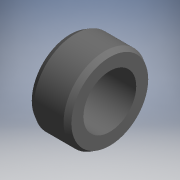
# Autodesk Inventor part: 189652 ZBH-5
Saved by Autodesk Inventor 2017.3 (Build 213256000, 256)
## iProperties
Part Number: 189652 ZBH-5
Material: Generic
Catalog Web Link: www.cadenas.de
Description: ZBH-centring sleeve
Vendor: FESTO
Document SubType Name: Modeling
Designer: partserver
Manufacturer: FESTO
Mass: 0.0270246 g
Surface Area: 0.808396 cm^2
Volume: 0.0270246 cm^3
Density: 1 g/cm^3
Appearance: PSOLRGB-128-128-128
Category: PARTsolutions
Company: FESTO
Title: 189652 ZBH-5
Author: Cadenas PARTsolutions
Comments: centring sleeve
PSOL_IDENT_0: {$CADENAS_DATA\23d-libs\festo\parts\z\zbh\zbh.prj},161 {VTYP=3D},{NB=189652 ZBH-5},{LINA=189652 ZBH-
PSOL_IDENT_1: 5},{NN=ZBH},{DATE=24.04.2020 12:36:33},{GEOMDATE=24.04.2020 12:01:39},{VERSION=},{LINEID=10},{WBVAR=
PSOL_IDENT_2: },{WBNUMERIC=}  {NB=189652 ZBH-5},{LINA=189652 ZBH-5},{KT=DUMMY},{TNR=189652},{TYP=ZBH-5},{B1=2.400}
PSOL_IDENT_3: ,{D1=5.000},{D2=3.200},{CNSMASSEXACT=0.000}
NB: 189652 ZBH-5
NN: ZBH
NT: centring sleeve
NBSYN: $TNR. $TYP.
LINA: 189652 ZBH-5
CATALOG: Festo
TNR: 189652
TYP: ZBH-5
B1: 2.4
D1: 5
D2: 3.2
CNSMASSEXACT: 0
SUPPLIER: FESTO
ARTICLENO: 189652 ZBH-5
BOMINFO: 189652 ZBH-5
CREATOR: CADENAS GmbH
Autodesk Inventor part; units mm, degrees
sketch "Sketch_1" plane through (0, 0, 0) normal (0, 0, 1) x (1, 0, 0)
  line L0 (2.4, 0) -> (0, 0)
  line L1 (0, 1.6) -> (2.4, 1.6)
  line L2 (2.4, 1.6) -> (2.4, 2.3268)
  line L3 (2.4, 2.3268) -> (2.1, 2.5)
  line L4 (2.1, 2.5) -> (0.3, 2.5)
  line L5 (0.3, 2.5) -> (0, 2.3268)
  line L6 (0, 2.3268) -> (0, 1.6)
  constraints: 14 end point
revolve "Revolution1" add sketch "Sketch_1" angle 360 about axis through (2.4, 0, 0) along (-1, 0, 0)
ref_plane "anbau_XY" through (0, 0, 0) normal (1, 0, 0) x (0, 0, -1)
ref_plane "anbau_YZ" through (0, 0, 0) normal (0, 0, -1) x (0, 1, 0)
ref_plane "anbau_ZX" through (0, 0, 0) normal (0, 1, 0) x (1, 0, 0)
ref_plane "insert_XY" through (0, 0, 0) normal (1, 0, 0) x (0, 0, -1)
ref_plane "insert_YZ" through (0, 0, 0) normal (0, 0, -1) x (0, 1, 0)
ref_plane "insert_ZX" through (0, 0, 0) normal (0, 1, 0) x (1, 0, 0)
ref_plane "schraube_punkt_XY" through (2.4, 0, 0) normal (1, 0, 0) x (0, 0, -1)
ref_plane "schraube_punkt_YZ" through (2.4, 0, 0) normal (0, 0, -1) x (0, 1, 0)
ref_plane "schraube_punkt_ZX" through (2.4, 0, 0) normal (0, 1, 0) x (1, 0, 0)
body "Solid1"
